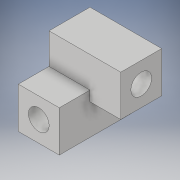
# Autodesk Inventor part: cam_holder_angle_part
Saved by Autodesk Inventor 2019 (Build 230136000, 136)
## iProperties
Created: 2024-08-06
Part Number: cam_holder_angle_part
Material: Generisch
Document SubType Name: Modeling
Designer: nic
Density: 1 g/cm^3
Appearance: Vorgabe
Author: nic
Autodesk Inventor part; units mm, degrees
ref_plane "YZ Plane" through (0, 0, 0) normal (1, 0, 0) x (0, 1, 0)
ref_plane "XZ Plane" through (0, 0, 0) normal (0, 1, 0) x (-1, 0, 0)
ref_plane "XY Plane" through (0, 0, 0) normal (0, 0, 1) x (1, 0, 0)
sketch "Skizze12" plane through (0, 0, 0) normal (0, 0, 1) x (1, 0, 0)
  circle A0 centre (0, 0) radius 10.1
  line L0 (-20, 20) -> (20, 20)
  line L1 (20, 20) -> (20, -20)
  line L2 (20, -20) -> (-20, -20)
  line L3 (-20, -20) -> (-20, 20)
  line L4 (-20, 20) -> (20, -20) construction
  line L5 (20, 20) -> (-20, -20) construction
  dimension "d59" = 20.2
  dimension "d60" = 40
  dimension "d61" = 40
  constraints: 12 end point, 2 midpoint, 2 parallel, 1 centre point, 1 coincident, 1 horizontal, 1 perpendicular
  measures "d59" diameter of A0
  measures "d60" distance of L1.end L2.end
  measures "d61" distance of L0.end L1.end
extrude "Extrusion10" add sketch "Skizze12" along normal blind 70
sketch "Skizze13" plane through (-20, -20, 0) normal (-1, 0, 0) x (0, 0, 1)
  line L0 (70, 30.1) -> (70, 9.9) projected
  line L1 (0, 9.9) -> (0, 30.1) projected
  line L2 (0, 30.1) -> (40, 30.1)
  line L3 (40, 30.1) -> (40, 70.1)
  line L4 (40, 70.1) -> (0, 70.1)
  line L5 (0, 70.1) -> (0, 30.1)
  circle A0 centre (20, 50.1) radius 10.1
  point P0 (0, 20)
  dimension "d64" = 40
  dimension "d65" = 40
  dimension "d66" = 20.2
  constraints: 8 end point, 2 parallel, 1 centre point, 1 horizontal, 1 perpendicular
  measures "d64" distance of L4.end L3.end
  measures "d65" distance of L3.end L2.end
  measures "d66" diameter of A0
extrude "Extrusion11" add sketch "Skizze13" against normal blind 70
